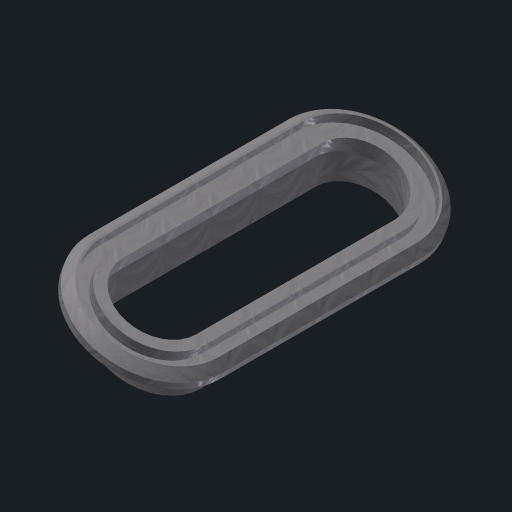
# Autodesk Inventor part: COMPUERTA_PLASTICO
Saved by Autodesk Inventor 2024.3 (Build 283343000, 343)
## iProperties
Created: 2024-07-04
Part Number: COMPUERTA_PLASTICO
Material: Steel, Mild, Welded
Document SubType Name: Modeling
Designer: Niler
Density: 7.85 g/cm^3
Appearance: Weld - Steel Mild
Author: Niler
Autodesk Inventor part; units mm, degrees
ref_plane "YZ Plane" through (0, 0, 0) normal (1, 0, 0) x (0, 1, 0)
ref_plane "XZ Plane" through (0, 0, 0) normal (0, 1, 0) x (-1, 0, 0)
ref_plane "XY Plane" through (0, 0, 0) normal (0, 0, 1) x (1, 0, 0)
sketch "Sketch1" plane through (0, 0, 0) normal (0, 1, 0) x (-1, 0, 0)
  line L0 (-101.5312, 175) -> (101.5312, 175)
  line L1 (101.5312, 175) -> (101.5312, -175)
  line L2 (101.5312, -175) -> (-101.5312, -175)
  line L3 (-101.5312, -175) -> (-101.5312, 175)
  line L4 (-101.5312, 175) -> (101.5312, -175) construction
  line L5 (101.5312, 175) -> (-101.5312, -175) construction
  point P0 (0, 0)
  dimension "d2" = 350
  constraints: 12 end point, 2 midpoint, 2 parallel, 1 horizontal, 1 perpendicular
  measures "d2" distance of L0.end L1.end
extrude "Extrusion1" add sketch "Sketch1" against normal blind 150
sketch "Sketch3" plane through (-101.5312, 0, 175) normal (0, 0, 1) x (-1, 0, 0)
  line L0 (0, 0) -> (-203.0624, 0) projected
  line L1 (-203.0624, 0) -> (-203.0624, 150) projected
  line L2 (-203.0624, 150) -> (0, 150) projected
  line L3 (0, 0) -> (0, 150) projected
  line L4 (0, 150) -> (-48.8156, 150)
  line L5 (0, 0) -> (47.3608, 0)
  line L6 (0, 0) -> (-203.0624, 81.2192)
  point P0 (-101.5312, 0)
  dimension "d7" = 158.2
  constraints: 6 end point, 2 horizontal, 1 point on line
  measures "d7" angle of L5 L6
extrude "Extrusion2" cut sketch "Sketch3" against normal through all contours L0 L1 L6
sketch "Sketch5" plane through (-101.5312, -150, 175) normal (0, 0, 1) x (1, 0, 0)
  line L0 (203.0624, 68.7808) -> (0, 150) projected
  line L1 (203.0624, 44.0093) -> (0, 125.2285)
  line L2 (0, 150) -> (0, 125.2285)
  line L3 (0, 150) -> (0, 0) projected
  line L4 (203.0624, 68.7808) -> (203.0624, 44.0093)
  line L5 (203.0624, 68.7808) -> (203.0624, 0) projected
  line L6 (203.0624, 0) -> (0, 0) projected
  point P0 (101.5312, 150)
  dimension "d13" = 23
  constraints: 8 end point, 1 parallel, 1 point on line, 1 vertical
  measures "d13" distance between parallel lines of L0 L1
extrude "Extrusion4" cut sketch "Sketch5" against normal through all contours L5 L6 L3 L1
sketch "Sketch4" plane through (0, 0, 0) normal (0, 1, 0) x (-1, 0, 0)
  line L0 (0, 95) -> (0, -95) construction
  line L1 (-45, 95) -> (-45, -95)
  line L2 (45, -95) -> (45, 95)
  arc A0 (45, 95) -> (-45, 95) centre (0, 95) ccw
  arc A1 (-45, -95) -> (45, -95) centre (0, -95) ccw
  line L3 (101.5312, -175) -> (-101.5312, -175) projected
  line L4 (101.5312, -175) -> (101.5312, 175) projected
  line L5 (-101.5312, 175) -> (101.5312, 175) projected
  line L6 (-101.5312, -175) -> (-101.5312, 175) projected
  line L7 (35, -95) -> (35, 95)
  arc A2 (35, 95) -> (-35, 95) centre (0, 95) ccw
  line L8 (-35, 95) -> (-35, -95)
  arc A3 (-35, -95) -> (35, -95) centre (0, -95) ccw
  point P0 (0, 0)
  dimension "d9" = 190
  dimension "d10" = 90
  dimension "d16" = 70
  constraints: 12 end point, 8 point on circle, 4 centre point, 4 tangent, 2 parallel, 1 midpoint, 1 vertical, 3 other
  measures "d9" distance of L0.start L0.end
  measures "d10" distance between parallel lines of L1 L2
  measures "d16" distance between parallel lines of L8 L7
extrude "Extrusion3" cut sketch "Sketch4" against normal through all
sketch "Sketch6" plane through (-45, -22.6109, 95) normal (0.3713678, 0.9284858, 0) x (0.9284858, -0.3713678, 0)
  line L0 (0, 190) -> (0, 0) projected
  ellipse E0 centre (48.466, 0) end of major axis (96.932, 0) minor radius 45 (0, 0) -> (96.932, 0) ccw projected
  line L1 (96.932, 0) -> (96.932, 190) projected
  ellipse E1 centre (48.466, 190) end of major axis (0, 190) minor radius 45 (96.932, 190) -> (0, 190) ccw projected
  line L2 (86.1618, 190) -> (86.1618, 0) projected
  ellipse E2 centre (48.466, 0) end of major axis (10.7702, 0) minor radius 35 (10.7702, 0) -> (86.1618, 0) ccw projected
  line L3 (10.7702, 0) -> (10.7702, 190) projected
  ellipse E3 centre (48.466, 190) end of major axis (86.1618, 190) minor radius 35 (86.1618, 190) -> (10.7702, 190) ccw projected
  line L4 (-20, 0) -> (-20, 190)
  line L5 (116.932, 190) -> (116.932, 0)
  spline S0 degree 5 poles (-20, 190) (-20, 192.7873) (-19.8429, 195.5746) (-19.5285, 198.3501) (-17.5293, 210.0569) (-12.7775, 221.1346) (-7.6435, 228.8473) (5.0656, 242.1963) (21.4308, 250.6892) (30.2419, 253.5617) (48.466, 256.4385) (66.6901, 253.5617) (75.5012, 250.6892) (91.8664, 242.1963) (104.5756, 228.8473) (109.7095, 221.1346) (114.4613, 210.0569) (116.4605, 198.3501) (116.7749, 195.5746) (116.932, 192.7873) (116.932, 190) knots 0 0 0 0 0 0 0.066461 0.066461 0.066461 0.282732 0.282732 0.282732 0.5 0.5 0.5 0.717268 0.717268 0.717268 0.933539 0.933539 0.933539 1 1 1 1 1 1
  spline S1 degree 5 poles (116.932, 0) (116.932, -2.7873) (116.7749, -5.5746) (116.4605, -8.3501) (114.4613, -20.0569) (109.7095, -31.1346) (104.5756, -38.8473) (91.8664, -52.1963) (75.5012, -60.6892) (66.6901, -63.5617) (48.466, -66.4385) (30.2419, -63.5617) (21.4308, -60.6892) (5.0656, -52.1963) (-7.6435, -38.8473) (-12.7775, -31.1346) (-17.5293, -20.0569) (-19.5285, -8.3501) (-19.8429, -5.5746) (-20, -2.7873) (-20, 0) knots 0 0 0 0 0 0 0.066461 0.066461 0.066461 0.282732 0.282732 0.282732 0.5 0.5 0.5 0.717268 0.717268 0.717268 0.933539 0.933539 0.933539 1 1 1 1 1 1
  point P0 (33.3849, 95)
  dimension "d17" = 20
  constraints: 4 end point, 3 parallel, 2 horizontal alignment, 8 other
  measures "d17" distance between parallel lines of L0 L4
extrude "Extrusion5" add sketch "Sketch6" along normal blind 15 contours E1 L1 E0 L0 | L4 S0 L5 S1
sketch "Sketch7" plane through (-39.4295, -8.6836, 95) normal (0.3713678, 0.9284858, 0) x (0.9284858, -0.3713678, 0)
  line L0 (116.932, 0) -> (116.932, 190) projected
  spline S0 degree 5 poles (116.932, 190) (116.932, 192.7873) (116.7749, 195.5746) (116.4605, 198.3501) (114.4613, 210.0569) (109.7095, 221.1346) (104.5756, 228.8473) (91.8664, 242.1963) (75.5012, 250.6892) (66.6901, 253.5617) (48.466, 256.4385) (30.2419, 253.5617) (21.4308, 250.6892) (5.0656, 242.1963) (-7.6435, 228.8473) (-12.7775, 221.1346) (-17.5293, 210.0569) (-19.5285, 198.3501) (-19.8429, 195.5746) (-20, 192.7873) (-20, 190) knots 0 0 0 0 0 0 0.066461 0.066461 0.066461 0.282732 0.282732 0.282732 0.5 0.5 0.5 0.717268 0.717268 0.717268 0.933539 0.933539 0.933539 1 1 1 1 1 1
  line L1 (-20, 190) -> (-20, 0) projected
  spline S1 degree 5 poles (-20, 0) (-20, -2.7873) (-19.8429, -5.5746) (-19.5285, -8.3501) (-17.5293, -20.0569) (-12.7775, -31.1346) (-7.6435, -38.8473) (5.0656, -52.1963) (21.4308, -60.6892) (30.2419, -63.5617) (48.466, -66.4385) (66.6901, -63.5617) (75.5012, -60.6892) (91.8664, -52.1963) (104.5756, -38.8473) (109.7095, -31.1346) (114.4613, -20.0569) (116.4605, -8.3501) (116.7749, -5.5746) (116.932, -2.7873) (116.932, 0) knots 0 0 0 0 0 0 0.066461 0.066461 0.066461 0.282732 0.282732 0.282732 0.5 0.5 0.5 0.717268 0.717268 0.717268 0.933539 0.933539 0.933539 1 1 1 1 1 1
  line L2 (10.7702, 0) -> (10.7702, 190) projected
  ellipse E0 centre (48.466, 190) end of major axis (10.7702, 190) minor radius 35 (86.1618, 190) -> (10.7702, 190) ccw projected
  line L3 (86.1618, 190) -> (86.1618, 0) projected
  ellipse E1 centre (48.466, 0) end of major axis (86.1618, 0) minor radius 35 (10.7702, 0) -> (86.1618, 0) ccw projected
  line L4 (106.932, 0) -> (106.932, 190)
  line L5 (-10, 190) -> (-10, 0)
  line L6 (96.1618, 0) -> (96.1618, 190)
  line L7 (0.7702, 190) -> (0.7702, 0)
  spline S2 degree 5 poles (106.932, 190.0001) (106.9319, 197.0563) (105.7307, 204.1143) (103.3237, 210.8942) (96.3256, 223.4758) (85.7343, 233.2374) (79.6784, 237.267) (66.5115, 243.4209) (52.1259, 245.5262) (44.8061, 245.5262) (30.4205, 243.4209) (17.2536, 237.267) (11.1977, 233.2374) (0.6064, 223.4758) (-6.3917, 210.8942) (-8.7987, 204.1143) (-9.9999, 197.0563) (-10, 190.0001) knots 0 0 0 0 0 0 0.197903 0.197903 0.197903 0.398748 0.398748 0.398748 0.601252 0.601252 0.601252 0.802098 0.802098 0.802098 1 1 1 1 1 1
  spline S3 degree 5 poles (-10, -0.0001) (-9.9999, -7.0563) (-8.7987, -14.1143) (-6.3917, -20.8942) (0.6064, -33.4758) (11.1977, -43.2374) (17.2536, -47.267) (30.4205, -53.4209) (44.8061, -55.5262) (52.1259, -55.5262) (66.5115, -53.4209) (79.6784, -47.267) (85.7343, -43.2374) (96.3256, -33.4758) (103.3237, -20.8942) (105.7307, -14.1143) (106.9319, -7.0563) (106.932, -0.0001) knots 0 0 0 0 0 0 0.197903 0.197903 0.197903 0.398748 0.398748 0.398748 0.601252 0.601252 0.601252 0.802097 0.802097 0.802097 1 1 1 1 1 1
  spline S4 degree 5 poles (96.1618, 190) (96.1618, 191.9179) (96.0537, 193.8357) (95.8373, 195.7454) (94.4556, 203.8347) (91.1648, 211.4879) (87.6047, 216.8191) (78.7576, 226.0938) (67.3691, 231.9934) (61.2077, 233.9967) (48.466, 236.0034) (35.7244, 233.9967) (29.5629, 231.9934) (18.1744, 226.0938) (9.3273, 216.8191) (5.7672, 211.4879) (2.4765, 203.8347) (1.0947, 195.7454) (0.8784, 193.8357) (0.7702, 191.9179) (0.7702, 190) knots 0 0 0 0 0 0 0.065841 0.065841 0.065841 0.281287 0.281287 0.281287 0.5 0.5 0.5 0.718713 0.718713 0.718713 0.934159 0.934159 0.934159 1 1 1 1 1 1
  spline S5 degree 5 poles (0.7702, 0) (0.7702, -1.9179) (0.8784, -3.8357) (1.0947, -5.7454) (2.4765, -13.8347) (5.7672, -21.4879) (9.3273, -26.8191) (18.1744, -36.0938) (29.5629, -41.9934) (35.7244, -43.9967) (48.466, -46.0034) (61.2077, -43.9967) (67.3691, -41.9934) (78.7576, -36.0938) (87.6047, -26.8191) (91.1648, -21.4879) (94.4556, -13.8347) (95.8373, -5.7454) (96.0537, -3.8357) (96.1618, -1.9179) (96.1618, 0) knots 0 0 0 0 0 0 0.065841 0.065841 0.065841 0.281287 0.281287 0.281287 0.5 0.5 0.5 0.718713 0.718713 0.718713 0.934159 0.934159 0.934159 1 1 1 1 1 1
  point P0 (33.3849, 95)
  dimension "d20" = 10
  dimension "d21" = 10
  constraints: 8 end point, 6 horizontal alignment, 6 parallel, 10 other
extrude "Extrusion6" cut sketch "Sketch7" against normal blind 10 contours S3 L5 S2 L4
chamfer "Chamfer1" distance 8 angle 45 4 edges at (5.5705, -26.6823, 160.0001) (69.1402, -52.1084, 0) (5.5705, -26.6823, -160.0001) (-57.9992, -1.2562, 0)
body "Solid1"
